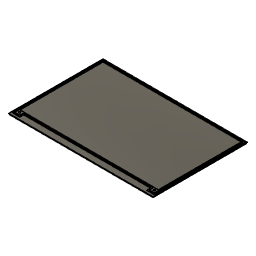
OpenBook_EBookReader_updated (Autodesk Fusion 360 archive; units mm, degrees)
design "Display"
Autodesk Fusion 360 part; units mm, degrees
sketch "Sketch1" plane through (0, 0, 0) normal (0, 0, 1) x (1, 0, 0)
  line L0 (-80, 90) -> (90.2, 90)
  line L1 (90.2, 90) -> (90.2, -21.2)
  line L2 (90.2, -21.2) -> (-80, -21.2)
  line L3 (-80, -21.2) -> (-80, 90)
  line L4 (-78.8, 88.8) -> (89, 88.8)
  line L5 (89, 88.8) -> (89, -18.29)
  line L6 (-78.8, -18.29) -> (-78.8, 88.8)
  line L7 (87.5, -16.79) -> (87.5, 87.3)
  line L8 (87.5, 87.3) -> (-77.3, 87.3)
  line L9 (-77.3, 87.3) -> (-77.3, -16.79)
  line L10 (-76.5, 86.5) -> (-76.5, -11.42)
  line L11 (-76.5, -11.42) -> (86.7, -11.42)
  line L12 (86.7, -11.42) -> (86.7, 86.5)
  line L13 (86.7, 86.5) -> (-76.5, 86.5)
  line L14 (-77.3, -16.79) -> (-71.3, -16.79)
  line L15 (-71.3, -13.22) -> (-71.3, -16.79)
  line L16 (-77.3, -16.79) -> (-71.3, -16.79)
  line L17 (87.5, -16.79) -> (81.5, -16.79)
  line L18 (-70.3, -12.22) -> (80.5, -12.22)
  line L19 (81.5, -13.22) -> (81.5, -16.79)
  line L20 (80, -18.29) -> (80, -14.72)
  line L21 (79, -13.72) -> (-68.8, -13.72)
  line L22 (-69.8, -18.29) -> (-69.8, -14.72)
  line L23 (89, -18.29) -> (80, -18.29)
  line L24 (-69.8, -18.29) -> (-78.8, -18.29)
  circle A0 centre (-74.3, -14.105) radius 1
  circle A1 centre (84.5, -14.105) radius 1
  arc A2 (-70.3, -12.22) -> (-71.3, -13.22) centre (-70.3, -13.22) ccw
  arc A3 (-68.8, -13.72) -> (-69.8, -14.72) centre (-68.8, -14.72) ccw
  arc A4 (81.5, -13.22) -> (80.5, -12.22) centre (80.5, -13.22) ccw
  arc A5 (80, -14.72) -> (79, -13.72) centre (79, -14.72) ccw
  dimension "d45" = 1
  constraint horizontal L0
  constraint perpendicular L0 L1
  constraint perpendicular L1 L2
  constraint perpendicular L0 L3
  constraint perpendicular L1 L4
  constraint perpendicular L0 L5
  constraint perpendicular L1 L23
  constraint perpendicular L4 L6
  constraint perpendicular L7 L16
  constraint perpendicular L6 L8
  constraint perpendicular L9 L16
  constraint perpendicular L7 L11
  constraint perpendicular L8 L12
  constraint perpendicular L10 L13
  constraint perpendicular L14 L15
  constraint perpendicular L7 L17
  constraint perpendicular L15 L18
  constraint perpendicular L20 L23
  constraint coincident L22.start L23
  constraint perpendicular L21 L22
  constraint collinear L23 L24
  constraint tangent L15 A2
  constraint tangent L18 A2
  constraint tangent L21 A3
  constraint tangent L22 A3
  constraint equal A2 A3
  constraint tangent L18 A4
  constraint tangent L19 A4
  constraint equal A2 A4
  constraint tangent L20 A5
  constraint tangent L21 A5
  constraint equal A2 A5
  measures "d45" radius of A2
extrude "Extrude1" add sketch "Sketch1" along normal blind 0.7 contours L0 L1 L2 L3
extrude "Extrude2" add sketch "Sketch1" along normal blind 1 contours L4 L5 L6 L20 L21 L22 L23 L24 A3 A5
extrude "Extrude3" add sketch "Sketch1" along normal blind 1.11 contours L7 L8 L9 L14 L15 L16 L17 L18 L19 A2 A4
extrude "Extrude4" add sketch "Sketch1" along normal blind 1.18 contours L10 L11 L12 L13
extrude "Extrude5" add sketch "Sketch1" along normal blind 1.18 contours A0
extrude "Extrude6" add sketch "Sketch1" along normal blind 1.18 contours A1

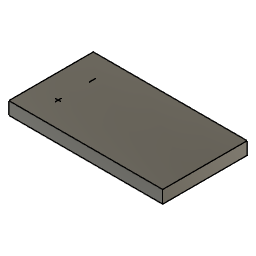
design "Battery"
Autodesk Fusion 360 part; units mm, degrees
sketch "Sketch1" plane through (0, 0, 0) normal (0, 0, 1) x (1, 0, 0)
  line L0 (-40, 20) -> (36.5, 20)
  line L1 (36.5, 20) -> (36.5, -22)
  line L2 (36.5, -22) -> (-40, -22)
  line L3 (-40, -22) -> (-40, 20)
  line L4 (-25, 10) -> (-25, 5)
  line L5 (-25, -5) -> (-25, -10)
  line L6 (-27.555614, -7.097658) -> (-22.555614, -7.097658)
  constraint horizontal L0
  constraint perpendicular L0 L1
  constraint perpendicular L1 L2
  constraint perpendicular L0 L3
  constraint perpendicular L0 L4
  constraint parallel L3 L5
  constraint perpendicular L5 L6
extrude "Extrude1" add sketch "Sketch1" along normal blind 6.3 contours L0 L1 L2 L3 picked at (-14.5, 6) makes body 1
sketch "Sketch2" plane through (0, 0, 6.3) normal (0, 0, 1) x (-1, 0, 0)
  line L0 (40, 22) -> (-36.5, 22)
  line L1 (-36.5, 22) -> (-36.5, -20)
  line L2 (-36.5, -20) -> (40, -20)
  line L3 (40, -20) -> (40, 22)
  line L4 (28, 10) -> (26, 10) construction
  line L5 (26, 10) -> (26, 8) construction
  line L6 (26, 8) -> (28, 8) construction
  line L7 (28, 8) -> (28, 10) construction
  line L8 (26, -7) -> (26, -9) construction
  line L9 (26, -9) -> (28, -9) construction
  line L10 (28, -9) -> (28, -7) construction
  line L11 (28, -7) -> (26, -7) construction
  dimension "d8" = 5
  dimension "d9" = 5
  text T0 "-" font "Arial" height 5 align centre top in box 2 x 2 at (26, -7) x (0, -1) y (1, 0) spacing 1 kerned
extrude "Extrude2" add sketch "Sketch2" sketch "Sketch2" along normal blind 0.01 contours L0 L1 L2 L3 picked at (-11, 8) of sketch 2 text T0 bodies 1
sketch "Sketch3" plane through (0, 0, 6.31) normal (0, 0, 1) x (-1, 0, 0)
  line L0 (40, -20) -> (40, 22)
  line L1 (40, 22) -> (-36.5, 22)
  line L2 (-36.5, 22) -> (-36.5, -20)
  line L3 (-36.5, -20) -> (40, -20)
  line L4 (28, 11) -> (27.986361, 11)
  line L5 (27.986361, 11) -> (27.986361, 8.000222)
  line L6 (27.986361, 8.000222) -> (28, 8.000222)
  line L7 (28, 8.000222) -> (28, 11)
  line L8 (29.232121, 9.482184) -> (26.699999, 9.482184)
  line L9 (26.699999, 9.482184) -> (26.699999, 9.5)
  line L10 (26.699999, 9.5) -> (29.232121, 9.5)
  line L11 (29.232121, 9.5) -> (29.232121, 9.482184)
  line L12 (27.96606, -9.007173) -> (28.017078, -9.007173)
  line L13 (28.017078, -9.007173) -> (28.017078, -5.945151)
  line L14 (28.017078, -5.945151) -> (27.96606, -5.945151)
  line L15 (27.96606, -5.945151) -> (27.96606, -9.007173)
  constraint horizontal L4
  constraint vertical L5
  constraint horizontal L6
  constraint vertical L7
  constraint horizontal L8
  constraint vertical L9
  constraint horizontal L10
  constraint vertical L11
  constraint horizontal L12
  constraint vertical L13
  constraint horizontal L14
  constraint vertical L15
extrude "Extrude3" add sketch "Sketch3" along normal blind 0.01 contours L12 L13 L14 L15 picked at (28.000072, -6.965825) bodies 1
extrude "Extrude4" add sketch "Sketch3" along normal blind 0.01 contours L5 L8 L9 L10 picked at (27.128787, 9.494061) bodies 1
extrude "Extrude5" add sketch "Sketch3" along normal blind 0.01 contours L7 L8 L10 L11 picked at (28.410707, 9.494061) bodies 1
extrude "Extrude6" add sketch "Sketch3" along normal blind 0.01 separate body contours L5 L6 L7 L8 picked at (27.990908, 8.988197) makes body 2
extrude "Extrude7" add sketch "Sketch3" along normal blind 0.01 separate body contours L4 L5 L7 L10 picked at (27.990908, 10.5) makes body 3
